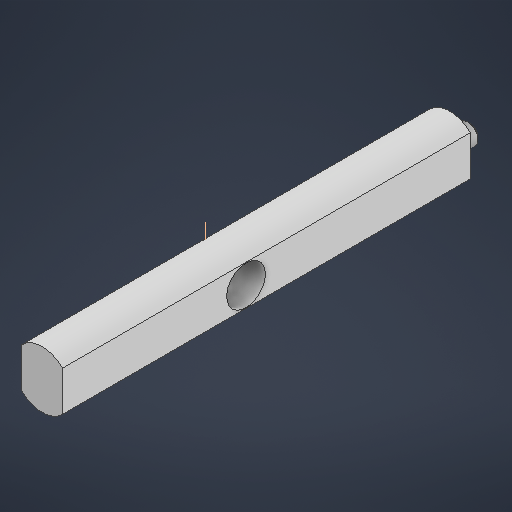
# Autodesk Inventor part: nozzle holder v1
Saved by Autodesk Inventor 2026.2 (Build 302298000, 298)
## iProperties
Created: 2026-01-17
Part Number: nozzle holder v1
Material: Generic
Document SubType Name: Modeling
Designer: User
Density: 1 g/cm^3
Appearance: Default
Author: User
Autodesk Inventor part; units mm, degrees
ref_plane "YZ Plane" through (0, 0, 0) normal (1, 0, 0) x (0, 1, 0)
ref_plane "XZ Plane" through (0, 0, 0) normal (0, 1, 0) x (-1, 0, 0)
ref_plane "XY Plane" through (0, 0, 0) normal (0, 0, 1) x (1, 0, 0)
sketch "Sketch1" plane through (0, 0, 0) normal (1, 0, 0) x (0, 1, 0)
  circle A0 centre (0, 0) radius 4.75
  line L0 (10, 45) -> (-10, 45)
  line L1 (10, 38) -> (-10, 38)
  line L2 (10, 45) -> (10, 38)
  line L3 (-10, 38) -> (-10, 45)
  line L4 (-4.75, 0) -> (-8.4137, 0)
  line L5 (-14, 0) -> (14, 0) projected
  line L6 (10, -55) -> (-10, -55)
  line L7 (-10, -55) -> (-10, -48)
  line L8 (-10, -48) -> (10, -48)
  line L9 (10, -48) -> (10, -55)
  line L10 (10, 38) -> (10, -48)
  line L11 (-10, -48) -> (-10, 38)
  point P0 (0, 45)
  point P1 (0, -55)
  dimension "d0" = 9.5
  dimension "d1" = 20
  dimension "d2" = 0
  dimension "d3" = 7
  dimension "d4" = 45
  dimension "d8" = 20
  dimension "d9" = 7
  dimension "d10" = 0
  dimension "d11" = 55
  constraints: 22 end point, 3 horizontal, 3 parallel, 2 midpoint, 2 perpendicular, 1 coincident, 1 horizontal alignment, 1 vertical, 2 other
  measures "d1" distance of L0.start L0.end
  measures "d2" horizontal distance of point (0, 45) point (0, 0)
  measures "d3" distance between parallel lines of L0 L1
  measures "d4" distance from line of L0 point (0, 0)
  measures "d8" distance of L7.end L8.end
  measures "d9" distance of L6.end L7.end
  measures "d10" horizontal distance of point (0, 0) point (0, -55)
  measures "d11" distance from line of point (0, 0) L6
extrude "Extrusion1" add sketch "Sketch1" along normal blind 10 contours L5 L10 L8 L11 L4 A0 | A0 L4 L5 L11 L1 L10 | L1 L3 L0 L2 | L9 L6 L7 L8
sketch "Sketch2" plane through (0, -10, -55) normal (0, 0, -1) x (-1, 0, 0)
  circle A0 centre (-5, 10) radius 2.475
  point P0 (0, 10)
  dimension "d12" = 4.95
  constraints: 1 centre point
  measures "d12" diameter of A0
extrude "Extrusion2" add sketch "Sketch2" along normal blind 4.9
chamfer "Chamfer1" distance 0.5 angle 45 1 edges at (7.475, 0, -59.9)
sketch "Sketch3" plane through (0, -10, -55) normal (0, 0, -1) x (-1, 0, 0)
  circle A0 centre (-5, 10) radius 2.475 projected
  circle A1 centre (-5, 10) radius 7
  circle A2 centre (-5, 10) radius 17.4724
  point P0 (0, 10)
  dimension "d18" = 14
  constraints: 2 centre point, 2 coincident
  measures "d18" diameter of A1
extrude "Extrusion3" cut sketch "Sketch3" against normal through all contours A2
body "Solid1"
